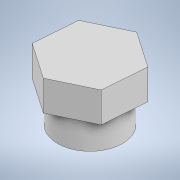
# Autodesk Inventor part: pieza1
Saved by Autodesk Inventor 2021 (Build 250183000, 183)
## iProperties
Created: 2023-05-09
Part Number: pieza1
Material: Generic
Document SubType Name: Modeling
Designer: assman
Density: 1 g/cm^3
Appearance: Default
Author: assman
Autodesk Inventor part; units mm, degrees
ref_plane "YZ Plane" through (0, 0, 0) normal (1, 0, 0) x (0, 1, 0)
ref_plane "XZ Plane" through (0, 0, 0) normal (0, 1, 0) x (-1, 0, 0)
ref_plane "XY Plane" through (0, 0, 0) normal (0, 0, 1) x (1, 0, 0)
sketch "Sketch1" plane through (0, 0, 0) normal (0, 1, 0) x (-1, 0, 0)
  circle A0 centre (0, 0) radius 10.7576
  constraints: 1 centre point, 1 coincident
extrude "Extrusion1" add sketch "Sketch1" along normal blind 10
sketch "Sketch2" plane through (0, 10, 0) normal (0, 1, 0) x (1, 0, 0)
  circle A0 centre (0, 0) radius 10.7576 projected
  circle A1 centre (0, 0) radius 2.9303
  constraints: 1 centre point, 1 coincident
extrude "Extrusion2" cut sketch "Sketch2" against normal blind 10 contours A1
sketch "Sketch3" plane through (0, 10, 0) normal (0, 1, 0) x (1, 0, 0)
  line L0 (11.8466, -8.1445) -> (-1.1301, -14.3317)
  line L1 (-1.1301, -14.3317) -> (-12.9767, -6.1872)
  line L2 (-12.9767, -6.1872) -> (-11.8466, 8.1445)
  line L3 (-11.8466, 8.1445) -> (1.1301, 14.3317)
  line L4 (1.1301, 14.3317) -> (12.9767, 6.1872)
  line L5 (12.9767, 6.1872) -> (11.8466, -8.1445)
  point P0 (0, 0)
  point P1 (0, 0)
  constraints: 12 end point, 1 coincident, 13 other
extrude "Extrusion3" add sketch "Sketch3" along normal blind 10
body "Solid1"
